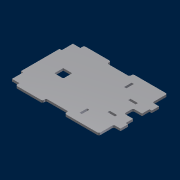
# Autodesk Inventor part: OpenROV_Dev_EChassis_Main_Plate
Saved by Autodesk Inventor 2012 (Build 160160000, 160)
## iProperties
Created: 2012-08-06
Part Number: OpenROV_Dev_EChassis_Main_Plate
Material: Default
Document SubType Name: Modeling
Designer: user
Density: 1 g/cm^3
Author: user
Autodesk Inventor part; units mm, degrees
ref_plane "YZ Plane" through (0, 0, 0) normal (1, 0, 0) x (0, 1, 0)
ref_plane "XZ Plane" through (0, 0, 0) normal (0, 1, 0) x (-1, 0, 0)
ref_plane "XY Plane" through (0, 0, 0) normal (0, 0, 1) x (1, 0, 0)
sketch "Sketch1" plane through (0, 0, 0) normal (0, 0, 1) x (1, 0, 0)
  line L0 (134, 62) -> (131, 62)
  line L1 (131, 30) -> (134, 30)
  line L2 (134, 20) -> (134, 30)
  line L3 (134, 62) -> (134, 72)
  line L4 (3, 87) -> (3, 72)
  line L5 (3, 72) -> (0, 72)
  line L6 (0, 20) -> (3, 20)
  line L7 (3, 20) -> (3, 5)
  line L8 (0, 72) -> (0, 20)
  line L9 (131, 52) -> (121, 52)
  line L10 (119, 50) -> (119, 42)
  line L11 (121, 40) -> (131, 40)
  line L12 (131, 62) -> (131, 52)
  line L13 (131, 40) -> (131, 30)
  line L14 (106, 61.5) -> (116, 61.5)
  line L15 (116, 61.5) -> (116, 58.5)
  line L16 (116, 58.5) -> (106, 58.5)
  line L17 (106, 58.5) -> (106, 61.5)
  line L18 (106, 33.5) -> (116, 33.5)
  line L19 (116, 33.5) -> (116, 30.5)
  line L20 (116, 30.5) -> (106, 30.5)
  line L21 (106, 30.5) -> (106, 33.5)
  line L22 (88, 81) -> (91, 81)
  line L23 (91, 81) -> (91, 71)
  line L24 (91, 71) -> (88, 71)
  line L25 (88, 71) -> (88, 81)
  line L26 (88, 21) -> (91, 21)
  line L27 (91, 21) -> (91, 11)
  line L28 (91, 11) -> (88, 11)
  line L29 (88, 11) -> (88, 21)
  line L30 (134, 20) -> (127, 20)
  line L31 (125, 2) -> (125, 18)
  line L32 (134, 72) -> (127, 72)
  line L33 (125, 90) -> (125, 74)
  line L34 (49, 90) -> (49, 89)
  line L35 (51, 87) -> (77, 87)
  line L36 (79, 89) -> (79, 90)
  line L37 (123, 92) -> (81, 92)
  line L38 (49, 2) -> (49, 3)
  line L39 (51, 5) -> (77, 5)
  line L40 (79, 3) -> (79, 2)
  line L41 (81, 0) -> (123, 0)
  arc A0 (49, 90) -> (47, 92) centre (47, 90) ccw
  arc A1 (49, 89) -> (51, 87) centre (51, 89) ccw
  arc A2 (77, 87) -> (79, 89) centre (77, 89) ccw
  arc A3 (81, 92) -> (79, 90) centre (81, 90) ccw
  arc A4 (125, 74) -> (127, 72) centre (127, 74) ccw
  arc A5 (121, 52) -> (119, 50) centre (121, 50) ccw
  arc A6 (119, 42) -> (121, 40) centre (121, 42) ccw
  arc A7 (127, 20) -> (125, 18) centre (127, 18) ccw
  arc A8 (79, 2) -> (81, 0) centre (81, 2) ccw
  arc A9 (79, 3) -> (77, 5) centre (77, 3) ccw
  arc A10 (51, 5) -> (49, 3) centre (51, 3) ccw
  arc A11 (47, 0) -> (49, 2) centre (47, 2) ccw
  arc A12 (123, 0) -> (125, 2) centre (123, 2) ccw
  arc A13 (125, 90) -> (123, 92) centre (123, 90) ccw
  line L42 (3, 5) -> (13, 5)
  line L43 (13, 5) -> (13, 2)
  line L44 (15, 0) -> (47, 0)
  line L45 (3, 87) -> (13, 87)
  line L46 (13, 87) -> (13, 90)
  line L47 (47, 92) -> (15, 92)
  line L48 (26, 52) -> (36, 52)
  line L49 (37, 51) -> (37, 41)
  line L50 (36, 40) -> (26, 40)
  line L51 (25, 41) -> (25, 51)
  arc A14 (25, 41) -> (26, 40) centre (26, 41) ccw
  arc A15 (26, 52) -> (25, 51) centre (26, 51) ccw
  arc A16 (37, 51) -> (36, 52) centre (36, 51) ccw
  arc A17 (36, 40) -> (37, 41) centre (36, 41) ccw
  arc A18 (13, 2) -> (15, 0) centre (15, 2) ccw
  arc A19 (15, 92) -> (13, 90) centre (15, 90) ccw
  point P0 (0, 0)
  point P1 (125, 0)
  point P2 (125, 92)
  point P3 (119, 52)
  point P4 (119, 40)
  point P5 (125, 20)
  point P6 (125, 72)
  point P7 (49, 87)
  point P8 (79, 87)
  point P9 (79, 92)
  point P10 (49, 0)
  point P11 (49, 5)
  point P12 (79, 5)
  point P13 (79, 0)
  point P14 (13, 0)
  point P15 (13, 92)
  point P16 (25, 52)
  point P17 (37, 40)
  point P18 (37, 52)
  dimension "d6" = 52
  dimension "d8" = 10
  dimension "d12" = 10
  dimension "d14" = 3
  dimension "d15" = 3
  dimension "d19" = 12
  dimension "d20" = 12
  dimension "d22" = 10
  dimension "d24" = 10
  dimension "d26" = 10
  dimension "d27" = 10
  dimension "d28" = 3
  dimension "d29" = 3
  dimension "d30" = 25
  dimension "d32" = 15
  dimension "d33" = 3
  dimension "d34" = 10
  dimension "d35" = 10
  dimension "d36" = 3
  dimension "d46" = 40
  dimension "d47" = 20
  dimension "d48" = 9
  dimension "d51" = 3
  dimension "d67" = 46
  dimension "d69" = 30
  dimension "d70" = 30
  dimension "d74" = 46
  dimension "d76" = 122
  dimension "d77" = 2
  dimension "d78" = 2
  dimension "d79" = 3
  dimension "d80" = 128
  dimension "d81" = 40
  dimension "d90" = 12
  dimension "d91" = 12
  dimension "d92" = 25
  dimension "d95" = 40
  dimension "d96" = 1
  dimension "d99" = 9
  dimension "d102" = 82
  dimension "d103" = 5
  dimension "d104" = 5
  dimension "d105" = 2
  constraints: 104 end point, 40 point on circle, 40 tangent, 35 point on line, 32 perpendicular, 20 centre point, 18 parallel, 16 equal radius, 7 horizontal
  measures "d6" distance of L5.end L6.start
  measures "d8" distance of L0.start L3.end
  measures "d12" distance of L2.start L1.end
  measures "d14" distance of L6.start L6.end
  measures "d15" distance of L1.start L1.end
  measures "d19" distance between parallel lines of L11 L9
  measures "d20" distance of L9.start point (119, 52)
  measures "d22" distance of L11.end L1.start
  measures "d24" distance between parallel lines of L9 L0
  measures "d26" distance of L14.start L14.end
  measures "d27" distance of L18.start L18.end
  measures "d28" distance of L20.end L18.start
  measures "d29" distance of L16.end L14.start
  measures "d30" distance between parallel lines of L16 L18
  measures "d32" distance between parallel lines of L12 L15
  measures "d33" distance of L22.start L22.end
  measures "d34" distance of L24.end L22.start
  measures "d35" distance of L28.end L26.start
  measures "d36" distance of L26.start L26.end
  measures "d46" distance between parallel lines of L13 L27
  measures "d47" distance of point (125, 0) point (125, 20)
  measures "d48" distance of L2.start point (125, 20)
  measures "d51" distance of L0.start L0.end
  measures "d67" distance between parallel lines of L4 L34
  measures "d69" distance between parallel lines of L36 L34
  measures "d70" distance between parallel lines of L40 L38
  measures "d74" distance between parallel lines of L7 L38
  measures "d76" distance between parallel lines of L7 L31
  measures "d77" radius of A0
  measures "d78" radius of A12
  measures "d79" distance between parallel lines of L4 L8
  measures "d80" distance between parallel lines of L12 L4
  measures "d81" distance between parallel lines of L12 L23
  measures "d90" distance of point (25, 52) point (37, 52)
  measures "d91" distance of point (37, 52) point (37, 40)
  measures "d92" distance between parallel lines of L8 L51
  measures "d95" distance between parallel lines of L47 L48
  measures "d96" radius of A14
  measures "d99" distance between parallel lines of L33 L3
  measures "d102" distance between parallel lines of L45 L42
  measures "d103" distance of L42.end point (13, 0)
  measures "d104" distance of L45.end point (13, 92)
  measures "d105" radius of A18
extrude "Extrusion6" add sketch "Sketch1" along normal blind 3
body "Solid6"
